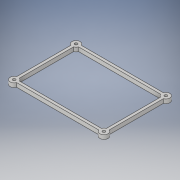
# Autodesk Inventor part: soporte_placa_separador
Saved by Autodesk Inventor 2019 (Build 230136000, 136)
## iProperties
Created: 2020-08-10
Part Number: soporte_placa_separador
Material: Generic
Document SubType Name: Modeling
Designer: Hugo Albarracin
Density: 1 g/cm^3
Appearance: Default
Author: Hugo Albarracin
Autodesk Inventor part; units mm, degrees
ref_plane "YZ Plane" through (0, 0, 0) normal (1, 0, 0) x (0, 1, 0)
ref_plane "XZ Plane" through (0, 0, 0) normal (0, 1, 0) x (-1, 0, 0)
ref_plane "XY Plane" through (0, 0, 0) normal (0, 0, 1) x (1, 0, 0)
sketch "Sketch1" plane through (0, 0, 0) normal (0, 1, 0) x (-1, 0, 0)
  line L0 (-33, 22.75) -> (33, 22.75) construction
  line L1 (33, 22.75) -> (33, -22.75) construction
  line L2 (33, -22.75) -> (-33, -22.75) construction
  line L3 (-33, -22.75) -> (-33, 22.75) construction
  line L4 (-33, 22.75) -> (33, -22.75) construction
  line L5 (33, 22.75) -> (-33, -22.75) construction
  line L6 (32, -21.75) -> (32, 21.75)
  line L7 (32, 21.75) -> (-32, 21.75)
  line L8 (-32, 21.75) -> (-32, -21.75)
  line L9 (-32, -21.75) -> (32, -21.75)
  line L10 (34, -23.75) -> (34, 23.75)
  line L11 (34, 23.75) -> (-34, 23.75)
  line L12 (-34, 23.75) -> (-34, -23.75)
  line L13 (-34, -23.75) -> (34, -23.75)
  point P0 (0, 0)
  dimension "d0" = 45.5
  dimension "d1" = 66
  dimension "d18" = 1
  dimension "d19" = 1
  constraints: 28 end point, 6 parallel, 3 perpendicular, 2 midpoint, 1 horizontal, 6 other
  measures "d0" distance of L0.end L1.end
  measures "d1" distance of L1.end L2.end
  measures "d18" distance between parallel lines of L1 L10
  measures "d19" distance between parallel lines of L6 L1
extrude "Extrusion1" add sketch "Sketch1" along normal blind 3
sketch "Sketch4" plane through (0, 3, 0) normal (0, 1, 0) x (1, 0, 0)
  line L0 (-32, -21.75) -> (-32, 21.75) construction
  line L1 (-34, 23.75) -> (-32, 21.75) construction
  line L2 (33, -22.75) -> (-33, -22.75) construction
  line L3 (-33, -22.75) -> (-33, 22.75) construction
  line L4 (-33, 22.75) -> (33, 22.75) construction
  line L5 (33, 22.75) -> (33, -22.75) construction
  line L6 (33, -22.75) -> (-33, 22.75) construction
  line L7 (-33, -22.75) -> (33, 22.75) construction
  circle A0 centre (-33, 22.75) radius 3
  circle A1 centre (33, 22.75) radius 3
  circle A2 centre (-33, -22.75) radius 3
  circle A3 centre (33, -22.75) radius 3
  point P0 (0, 0)
  dimension "d20" = 6
  dimension "d21" = 6
  dimension "d22" = 6
  dimension "d23" = 6
  constraints: 14 end point, 4 centre point, 4 coincident, 3 midpoint, 2 parallel, 1 horizontal, 1 perpendicular
  measures "d20" diameter of A0
  measures "d21" diameter of A1
  measures "d22" diameter of A2
  measures "d23" diameter of A3
extrude "Extrusion3" add sketch "Sketch4" against normal up to surface (3 mm away)
sketch "Sketch5" plane through (0, 3, 0) normal (0, 1, 0) x (1, 0, 0)
  line L0 (-30.1716, -23.75) -> (30.1716, -23.75) projected
  arc A0 (30.1716, -23.75) -> (34, -19.9216) centre (33, -22.75) ccw projected
  line L1 (34, -19.9216) -> (34, 19.9216) projected
  arc A1 (34, 19.9216) -> (30.1716, 23.75) centre (33, 22.75) ccw projected
  line L2 (30.1716, 23.75) -> (-30.1716, 23.75) projected
  arc A2 (-30.1716, 23.75) -> (-34, 19.9216) centre (-33, 22.75) ccw projected
  line L3 (-34, 19.9216) -> (-34, -19.9216) projected
  arc A3 (-34, -19.9216) -> (-30.1716, -23.75) centre (-33, -22.75) ccw projected
  arc A4 (-30.1716, -21.75) -> (-32, -19.9216) centre (-33, -22.75) ccw projected
  line L4 (-32, -19.9216) -> (-32, 19.9216) projected
  arc A5 (-32, 19.9216) -> (-30.1716, 21.75) centre (-33, 22.75) ccw projected
  line L5 (-30.1716, 21.75) -> (30.1716, 21.75) projected
  arc A6 (30.1716, 21.75) -> (32, 19.9216) centre (33, 22.75) ccw projected
  line L6 (32, 19.9216) -> (32, -19.9216) projected
  arc A7 (32, -19.9216) -> (30.1716, -21.75) centre (33, -22.75) ccw projected
  line L7 (30.1716, -21.75) -> (-30.1716, -21.75) projected
  point P0 (0, 0)
hole "Hole2" at (-33, 3, -22.75) at (33, 3, -22.75) at (-33, 3, 22.75) at (33, 3, 22.75) direction (0, -1, 0) diameter 2 depth 25 tip angle 118
equation "\"d18\" = d19"
equation "\"d21\" = d20"
equation "\"d22\" = d20"
equation "\"d23\" = d20"
body "Solid1"
